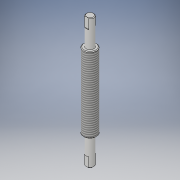
# Autodesk Inventor part: Вал
Saved by Autodesk Inventor 2019 (Build 230136000, 136)
## iProperties
Created: 2021-03-17
Part Number: Вал
Material: Типовые
Document SubType Name: Modeling
Designer: Петров Иван
Density: 1 g/cm^3
Appearance: По умолчанию
Mass: 5.69839 g
Surface Area: 27.3708 cm^2
Volume: 5.69839 cm^3
Author: Петров Иван
Autodesk Inventor part; units mm, degrees
ref_plane "YZ Plane" through (0, 0, 0) normal (1, 0, 0) x (0, 1, 0)
ref_plane "XZ Plane" through (0, 0, 0) normal (0, 1, 0) x (-1, 0, 0)
ref_plane "XY Plane" through (0, 0, 0) normal (0, 0, 1) x (1, 0, 0)
sketch "Sketch1" plane through (0, 0, 0) normal (0, 1, 0) x (-1, 0, 0)
  circle A0 centre (0, 0) radius 3
  dimension "d0" = 6
  constraints: 1 centre point, 1 coincident
  measures "d0" diameter of A0
extrude "Extrusion1" add sketch "Sketch1" along normal blind 100
chamfer "Chamfer1" distance 0.5 angle 45 2 edges at (3, 100, 0) (3, 0, 0)
sketch "Sketch3" plane through (0, 100, 0) normal (0, 1, 0) x (1, 0, 0)
  circle A0 centre (0, 0) radius 3 projected
  line L0 (-1.6583, -2.5) -> (1.6583, -2.5)
  dimension "d16" = 2.5
  constraints: 2 end point, 2 point on circle, 1 horizontal
  measures "d16" distance from line of point (0, 0) L0
extrude "Extrusion3" cut sketch "Sketch3" against normal blind 7.5 contours L0 A0 picked at (-0.3442, -2.6056)
mirror "Mirror1" about plane through (0, 0, 0) normal (0, 0, 1) of "Extrusion3"
ref_plane "Work Plane3" through (0, 50, 0) normal (0, -1, 0) x (1, 0, 0)
mirror "Mirror2" about plane through (0, 50, 0) normal (0, -1, 0) of "Extrusion3", "Mirror1"
sketch "Sketch4" plane through (0, 50, 0) normal (0, -1, 0) x (1, 0, 0)
  circle A0 centre (0, 0) radius 5
  dimension "d20" = 10
  constraints: 1 centre point, 1 coincident
  measures "d20" diameter of A0
extrude "Extrusion4" add sketch "Sketch4" along normal mid plane 58
chamfer "Chamfer3" distance 0.5 angle 45 2 edges at (-5, 21, 0) (-5, 79, 0)
thread "Thread3" size "M10x1.5" class "6g" standard "ANSI Metric M Profile" full length
body "Solid1"
